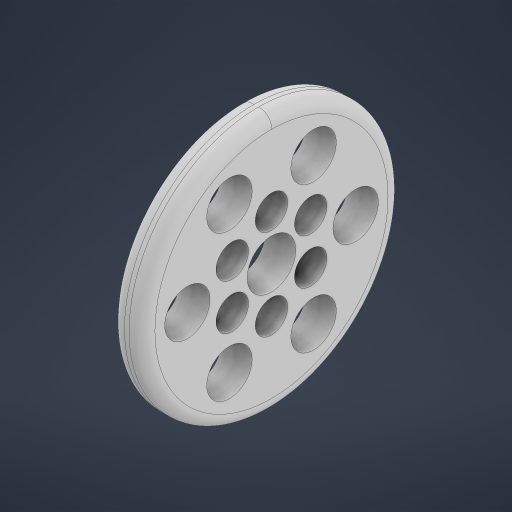
# Autodesk Inventor part: small_wheel
Saved by Autodesk Inventor 2024.2 (Build 282272000, 272)
## iProperties
Created: 2024-03-13
Part Number: small_wheel
Material: Generic
Document SubType Name: Modeling
Designer: jerem
Density: 1 g/cm^3
Appearance: Default
Author: jerem
## iProperties of the stored document small_wheel_3DPrint.ipt
Created: 2024-03-18
Part Number: small_wheel_3DPrint
Material: Generic
Document SubType Name: Modeling
Designer: jerem
Density: 1 g/cm^3
Appearance: Default
Author: jerem
Autodesk Inventor part; units mm, degrees
ref_plane "YZ Plane" through (0, 0, 0) normal (1, 0, 0) x (0, 1, 0)
ref_plane "XZ Plane" through (0, 0, 0) normal (0, 1, 0) x (-1, 0, 0)
ref_plane "XY Plane" through (0, 0, 0) normal (0, 0, 1) x (1, 0, 0)
sketch "Sketch2" plane through (0, 0, 0) normal (1, 0, 0) x (0, 1, 0)
  circle A0 centre (0, 0) radius 20
  circle A1 centre (0, 0) radius 3.75
  circle A2 centre (11.875, 0) radius 3.75
  line L0 (20, 0) -> (15.625, 0) construction
  line L1 (8.125, 0) -> (3.75, 0) construction
  line L2 (0, 0) -> (3.75, 0) construction
  circle A3 centre (0, 11.875) radius 3.75
  circle A4 centre (-11.875, 0) radius 3.75
  circle A5 centre (0, -11.875) radius 3.75
  circle A6 centre (8.3969, 8.3969) radius 3.75
  circle A7 centre (0, 11.875) radius 3.75
  circle A8 centre (-8.3969, 8.3969) radius 3.75
  circle A9 centre (-11.875, 0) radius 3.75
  circle A10 centre (-8.3969, -8.3969) radius 3.75
  circle A11 centre (0, -11.875) radius 3.75
  circle A12 centre (8.3969, -8.3969) radius 3.75
  point P0 (0, 15.625)
  point P1 (0, 8.125)
  point P2 (-15.625, 0)
  point P3 (-8.125, 0)
  point P4 (0, -15.625)
  point P5 (0, -8.125)
  point P6 (11.0485, 11.0485)
  point P7 (5.7452, 5.7452)
  point P8 (0, 15.625)
  point P9 (0, 8.125)
  point P10 (-11.0485, 11.0485)
  point P11 (-5.7452, 5.7452)
  point P12 (-15.625, 0)
  point P13 (-8.125, 0)
  point P14 (-11.0485, -11.0485)
  point P15 (-5.7452, -5.7452)
  point P16 (0, -15.625)
  point P17 (0, -8.125)
  point P18 (11.0485, -11.0485)
  point P19 (5.7452, -5.7452)
  dimension "d0" = 40
  dimension "d1" = 7.5
  dimension "d6" = 360
  dimension "d10" = 360
  dimension "d12" = 7.5
  constraints: 22 point on circle, 11 centre point, 6 end point, 2 coincident, 2 collinear, 2 horizontal alignment, 2 point on line, 1 horizontal, 1 line through centre, 54 other
  measures "d12" diameter of A2
extrude "Extrusion1" add sketch "Sketch2" along normal blind 4.7 contours A0 | A2 | A3 | A4 | A5 | A6 | A8 | A10 | A12
fillet "Fillet1" radius 2 2 edges at (4.7, -20, 0) (0, -20, 0) curvature continuous yes
sketch "Sketch3" plane through (4.7, 0, 0) normal (1, 0, 0) x (0, 0, -1)
  circle A0 centre (0, 7) radius 2.5
  circle A1 centre (-6.0622, 3.5) radius 2.5
  circle A2 centre (-6.0622, -3.5) radius 2.5
  circle A3 centre (0, -7) radius 2.5
  circle A4 centre (6.0622, -3.5) radius 2.5
  circle A5 centre (6.0622, 3.5) radius 2.5
  circle A6 centre (-6.5, 11.2583) radius 3.5
  line L0 (-6.5, 11.2583) -> (-6.0622, 3.5) construction
  line L1 (-6.5, 11.2583) -> (0, 7) construction
  circle A7 centre (-13, 0) radius 3.5
  circle A8 centre (-6.5, -11.2583) radius 3.5
  circle A9 centre (6.5, -11.2583) radius 3.5
  circle A10 centre (13, 0) radius 3.5
  circle A11 centre (6.5, 11.2583) radius 3.5
  point P0 (0, 0)
  dimension "d15" = 5
  dimension "d16" = 7
  dimension "d19" = 360
  dimension "d21" = 7
  dimension "d27" = 0
  dimension "d28" = 13
  dimension "d33" = 360
  constraints: 12 centre point, 4 end point, 1 equal length, 26 other
  measures "d15" diameter of A0
  measures "d16" distance of point (0, 0) L1.end
  measures "d21" diameter of A6
  measures "d27" horizontal distance of point (0, 0) L1.end
  measures "d28" distance of point (0, 0) L0.start
extrude "Extrusion2" cut sketch "Sketch3" against normal blind 4.7
body "Solid1"
